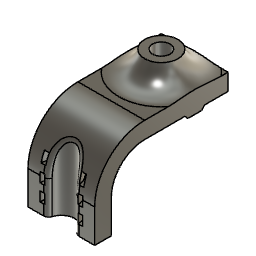
umbilical_support v3 (Autodesk Fusion 360 design; units mm, degrees)
Autodesk Fusion 360 part; units mm, degrees
note: some values were not read from the file. Set by a fixed rule: which sketch regions a step uses.
sketch "Esquisse1" plane through (0, 0, 0) normal (0, 0, 1) x (1, 0, 0)
  line L0 (-10, 0) -> (-10, 40)
  line L1 (-10, 40) -> (10, 40)
  line L2 (10, 40) -> (10, 0)
  line L3 (-10, 0) -> (10, 0) construction
  arc A0 (4, 0) -> (-4, 0) centre (0, 0) ccw
  line L4 (-4, 0) -> (-10, 0)
  line L5 (4, 0) -> (10, 0)
  line L6 (0, 40) -> (0, 0) construction
  circle A1 centre (0, 0) radius 10
  line L7 (-8.6603, 5) -> (-10, 5)
  line L8 (10, 5) -> (8.6603, 5)
  dimension "d1" = 8
  dimension "d2" = 20
  dimension "d3" = 40
  dimension "d21" = 20
  dimension "d24" = 5
  dimension "d25" = 5
  constraint coincident A0.centre L6.end
  constraint vertical L0
  constraint perpendicular L0 L1
  constraint perpendicular L1 L2
  constraint horizontal L3
  constraint coincident L3 A0.end
  constraint coincident L3 A0.start
  constraint midpoint L1 L6.start
  constraint vertical L6
  constraint coincident A0.centre L3
  constraint concentric A0 A1
  constraint coincident A1 L7.start
  constraint coincident L0 L7.end
  constraint perpendicular L0 L7
  constraint coincident L2 L8.start
  constraint coincident A1 L8.end
  constraint perpendicular L2 L8
  measures "d1" diameter of A0
  measures "d2" distance of L0.end L1.end
  measures "d3" distance of L1.end L2.end
  measures "d21" diameter of A1
  measures "d24" distance of L0.start L7.end
  measures "d25" distance of L2.end L8.start
extrude "Extrusion1" add sketch "Esquisse1" along normal blind 5 contours A0 L4 L5 A1 | L0 A1 L7 | L0 L1 L2 A1 L7 L8 | L2 A1 L8 picked at (6.5945, 4.4961)
extrude "Extrusion2" add sketch "Esquisse1" against normal blind 20 contours A0 L4 L5 A1 | L0 A1 L7 | L2 A1 L8 picked at (6.5945, 4.4961)
sketch "Esquisse2" plane through (-10, 0, 0) normal (-1, 0, 0) x (0, -1, 0)
  line L0 (-40, 0) -> (-5, 0)
  line L1 (0, -20) -> (0, 5)
  line L2 (0, 5) -> (-40, 5)
  line L3 (-40, 5) -> (-40, 0)
  line L4 (-33, 0) -> (-32, -1)
  line L5 (-32, -1) -> (-28, -1)
  line L6 (-28, -1) -> (-27, 0)
  line L7 (0, 0) -> (-40, 0)
  line L8 (-30, -1) -> (-30, 0) construction
  line L9 (-5, 0) -> (-5, -20)
  line L10 (-5, -20) -> (0, -20)
  dimension "d9" = 45
  dimension "d10" = 45
  dimension "d11" = 10
  dimension "d12" = 1
  dimension "d13" = 6
  constraint coincident L0 L4.start
  constraint parallel L0 L5
  constraint coincident L0 L6.end
  constraint midpoint L5 L8.start
  constraint coincident L7 L8.end
  constraint perpendicular L7 L8
  measures "d9" angle of L4 L7
  measures "d10" angle of L6 L7
  measures "d11" distance of L0.start L8.end
  measures "d12" distance of L5 L7
  measures "d13" distance of L4.start L6.end
extrude "Extrusion3" add sketch "Esquisse2" against normal up to surface (20 mm away) contours L0 L4 L5 L6 L7
sketch "Esquisse3" plane through (0, 0, 5) normal (0, 0, 1) x (-1, 0, 0)
  arc A0 (-4, 0) -> (4, 0) centre (0, 0) ccw
  line L0 (-4, 0) -> (-10, 0)
  line L1 (-10, 0) -> (-10, -40)
  line L2 (-10, -40) -> (10, -40)
  line L3 (10, -40) -> (10, 0)
  line L4 (10, 0) -> (4, 0)
  line L5 (0, -40) -> (0, -30) construction
  circle A1 centre (0, -30) radius 2.75
  circle A2 centre (0, -30) radius 5
  dimension "d16" = 5.5
  dimension "d17" = 10
  dimension "d18" = 10
  constraint midpoint L2 L5.start
  constraint perpendicular L2 L5
  constraint coincident L5.end A1.centre
  constraint concentric A1 A2
  measures "d16" diameter of A1
  measures "d17" distance of L5.start L5.end
  measures "d18" diameter of A2
sketch "Esquisse4" plane through (10, 0, 0) normal (1, 0, 0) x (0, 1, 0)
  line L0 (33, 0) -> (40, 0)
  line L1 (40, 0) -> (40, 5)
  line L2 (40, 5) -> (0, 5)
  line L3 (0, 5) -> (0, -20)
  line L4 (0, -20) -> (5, -20)
  line L5 (5, -20) -> (5, 0)
  line L6 (5, 0) -> (27, 0)
  line L7 (27, 0) -> (28, -1)
  line L8 (28, -1) -> (32, -1)
  line L9 (32, -1) -> (33, 0)
  circle A0 centre (15, -10) radius 10
  circle A1 centre (15, -10) radius 15
  dimension "d28" = 20
  constraint tangent L6 A0
  constraint tangent L5 A0
  constraint concentric A0 A1
  constraint tangent L3 A1
  measures "d28" diameter of A0
extrude "Extrusion5" add sketch "Esquisse4" against normal blind 20 contours L5 L6 A0
extrude "Extrusion6" cut sketch "Esquisse4" against normal blind 35 contours L2 L3 A1
fillet "Congé3" radius 1.5 3 edges at (-8.6603, 5, -15) (0, 10, -1.3397) (8.6603, 5, -15)
fillet "Congé4" radius 1.5 3 edges at (4, 0, -15) (0, 4, 0.198) (-4, 0, -15)
sketch "Esquisse5" plane through (0, 0, 0) normal (0, 1, 0) x (1, 0, 0)
  line L0 (5, 4) -> (6.4, 4)
  line L1 (6.4, 4) -> (6.4, 6.9)
  line L2 (6.4, 6.9) -> (5, 6.9)
  line L3 (5, 6.9) -> (5, 4)
  line L4 (5.7, 4) -> (5.7, 6.9) construction
  dimension "d37" = 1.4
  dimension "d38" = 2.9
  dimension "d40" = 4
  dimension "d42" = 5
  constraint horizontal L0
  constraint vertical L1
  constraint horizontal L2
  constraint vertical L3
  constraint midpoint L0 L4.start
  constraint midpoint L2 L4.end
  measures "d37" distance of L1.end L2.end
  measures "d38" distance of L0.end L1.end
  measures "d40" vertical distance of L4.start origin
  measures "d42" horizontal distance of origin L0.start
revolve "Révolution1" cut sketch "Esquisse5" angle 360 about axis through (0, 0, 1.75) along (0, 0, 1)
pattern_linear "Réseau R1" count 3 spacing 5 along (0, 0, -1) of "Révolution1"
sketch "Esquisse6" plane through (0, 0, 5) normal (0, 0, 1) x (-1, 0, 0)
  line L0 (10, -15) -> (-10, -15)
  line L1 (-10, -15) -> (-10, -40)
  line L2 (-10, -40) -> (10, -40)
  line L3 (10, -40) -> (10, -15)
  line L4 (0, -40) -> (0, -30) construction
  circle A0 centre (0, -30) radius 5
  circle A1 centre (0, -30) radius 2.625
  dimension "d47" = 5.25
  dimension "d48" = 10
  dimension "d49" = 10
  constraint midpoint L2 L4.start
  constraint perpendicular L2 L4
  constraint coincident L4.end A0.centre
  constraint concentric A0 A1
  measures "d47" diameter of A1
  measures "d48" diameter of A0
  measures "d49" distance of L4.start L4.end
extrude "Extrusion7" add sketch "Esquisse6" along normal blind 6 contours A0
extrude "Extrusion8" cut 1 faces at (0.1132, 31.9411, 5) along direction (0, 0, -1) blind 16
fillet "Congé5" radius 8 1 edges at (4.6616, 28.1919, 5)
equation "d37 = 0.9 mm + 0.5 mm"
equation "d38 = 2.40 mm + 0.5 mm"
